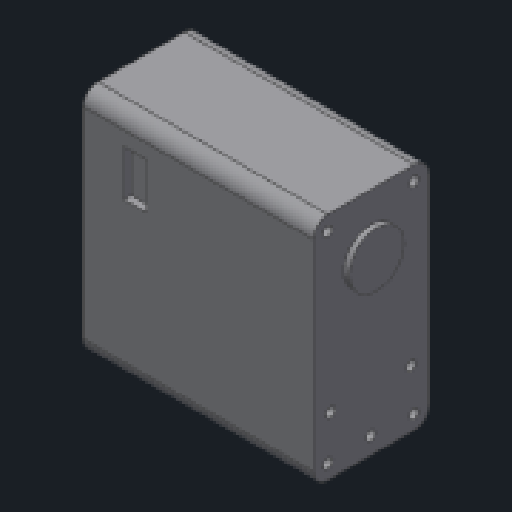
# Autodesk Inventor part: FeeTechSTS3025BL
Saved by Autodesk Inventor 2025.2 (Build 292293000, 293)
## iProperties
Created: 2025-07-25
Part Number: FeeTechSTS3025BL
Material: Generic
Document SubType Name: Modeling
Designer: valer
Density: 1 g/cm^3
Appearance: Default
Author: valer
Autodesk Inventor part; units mm, degrees
ref_plane "YZ Plane" through (0, 0, 0) normal (1, 0, 0) x (0, 1, 0)
ref_plane "XZ Plane" through (0, 0, 0) normal (0, 1, 0) x (-1, 0, 0)
ref_plane "XY Plane" through (0, 0, 0) normal (0, 0, 1) x (1, 0, 0)
sketch "Base" plane through (0, 0, 0) normal (0, 0, 1) x (1, 0, 0)
  line L0 (-20, 20) -> (20, 20)
  line L1 (20, 20) -> (20, -20)
  line L2 (20, -20) -> (-20, -20)
  line L3 (-20, -20) -> (-20, 20)
  line L4 (0, 20) -> (0, -20) construction
  point P0 (0, 0)
  point P1 (0, 0)
  dimension "d0" = 40
  dimension "d1" = 40
  constraints: 10 end point, 3 midpoint, 2 parallel, 1 coincident, 1 horizontal, 1 perpendicular
  measures "d0" distance of L0.start L0.end
  measures "d1" distance of L0.end L1.end
extrude "BaseFeature" add sketch "Base" along normal mid plane 20
sketch "Axis" plane through (20, -20, 10) normal (1, 0, 0) x (0, 0, -1)
  circle A0 centre (10, 30) radius 10 construction
  line L0 (20, 40) -> (0, 40) construction
  line L1 (0, 0) -> (0, 40) construction
  circle A1 centre (10, 30) radius 4.75
  line L2 (20, 40) -> (20, 0) projected
  point P0 (10, 20)
  dimension "d4" = 9.5
  constraints: 3 tangent, 2 centre point, 1 coincident
  measures "d4" diameter of A1
extrude "AxisFeature" add sketch "Axis" along normal blind 1
mirror "AxisMirrorFeature" about plane through (0, 0, 0) normal (1, 0, 0) of "AxisFeature"
sketch "Sketch3" plane through (0, 0, 10) normal (0, 0, 1) x (1, 0, 0)
  line L0 (-13, 15) -> (-9, 15)
  line L1 (-9, 15) -> (-9, 7)
  line L2 (-9, 7) -> (-13, 7)
  line L3 (-13, 7) -> (-13, 15)
  line L4 (20, 20) -> (-20, 20) projected
  line L5 (-20, 20) -> (-20, -20) projected
  point P0 (0, 0)
  point P1 (-11, 15)
  dimension "d7" = 8
  dimension "d8" = 4
  dimension "d9" = 5
  dimension "d10" = 7
  constraints: 8 end point, 2 parallel, 1 horizontal, 1 midpoint, 1 perpendicular
  measures "d7" distance of L0.end L1.end
  measures "d8" distance of L0.start L0.end
  measures "d9" distance from line of L4 point (-11, 15)
  measures "d10" distance between parallel lines of L5 L3
extrude "Extrusion3" cut sketch "Sketch3" against normal blind 1.3
fillet "Fillet1" radius 2.5 4 edges at (0, 20, 10) (0, -20, 10) (0, -20, -10) (0, 20, -10)
sketch "Sketch4" plane through (20, -17.5, 10) normal (1, 0, 0) x (0, 0, -1)
  arc A0 (2.5, 37.5) -> (0, 35) centre (2.5, 35) ccw projected
  arc A1 (20, 35) -> (17.5, 37.5) centre (17.5, 35) ccw projected
  arc A2 (0, 0) -> (2.5, -2.5) centre (2.5, 0) ccw projected
  arc A3 (17.5, -2.5) -> (20, 0) centre (17.5, 0) ccw projected
  circle A4 centre (2.5, 35) radius 0.85
  circle A5 centre (17.5, 35) radius 0.85
  circle A6 centre (2.5, 0) radius 0.85
  circle A7 centre (17.5, 0) radius 0.85
  point P0 (10, 17.5)
  dimension "d14" = 1.7
  constraints: 4 centre point, 4 coincident, 3 equal radius
  measures "d14" diameter of A4
extrude "Extrusion4" cut sketch "Sketch4" against normal blind 10
mirror "Mirror2" about plane through (0, 0, 0) normal (1, 0, 0) of "Extrusion4"
sketch "Sketch6" plane through (-20, -17.5, -10) normal (-1, 0, 0) x (0, 0, 1)
  circle A0 centre (17.5, 0) radius 0.85 construction
  circle A1 centre (2.5, 0) radius 0.85 construction
  line L0 (17.5, 0) -> (2.5, 0) construction
  line L1 (2.5, 0) -> (2.5, 15) construction
  line L2 (2.5, 15) -> (17.5, 15) construction
  line L3 (17.5, 15) -> (17.5, 0) construction
  circle A2 centre (17.5, 15) radius 0.85
  circle A3 centre (2.5, 15) radius 0.85
  point P0 (10, 17.5)
  dimension "d18" = 15
  constraints: 8 end point, 3 coincident, 2 centre point, 2 equal radius, 2 parallel, 2 perpendicular, 1 horizontal
  measures "d18" distance of L0.start L0.end
extrude "Extrusion5" cut sketch "Sketch6" against normal blind 10
sketch "Sketch7" plane through (20, -17.5, 10) normal (1, 0, 0) x (0, 0, -1)
  line L0 (0, 0) -> (0, 35) construction
  line L1 (20, 35) -> (20, 0) construction
  circle A0 centre (10, 7.5) radius 10 construction
  line L2 (17.5, -2.5) -> (2.5, -2.5) construction
  circle A1 centre (10, 7.5) radius 4 construction
  line L3 (10, 17.5) -> (10, -2.5) construction
  line L4 (0, 7.5) -> (20, 7.5) construction
  line L5 (10, 11.5) -> (10, 17.5) construction
  circle A2 centre (10, 14.5) radius 0.85
  line L6 (10, 3.5) -> (10, -2.5) construction
  line L7 (20, 0) -> (20, 35) projected
  circle A3 centre (10, 0.5) radius 0.85
  line L8 (0, 7.5) -> (6, 7.5) construction
  line L9 (14, 7.5) -> (20, 7.5) construction
  circle A4 centre (3, 7.5) radius 0.85
  circle A5 centre (17, 7.5) radius 0.85
  circle A6 centre (2.5, 0) radius 0.85 projected
  dimension "d21" = 8
  constraints: 12 end point, 6 centre point, 6 point on circle, 6 point on line, 5 midpoint, 4 equal radius, 3 tangent, 2 collinear, 1 coincident, 1 parallel
  measures "d21" diameter of A1
extrude "Extrusion6" cut sketch "Sketch7" against normal blind 10 contours A3 | A4 | A5
ref_plane "Work Plane1" through (0, 0, 0) normal (1, 0, 0) x (0, 1, 0)
body "Solid1"
